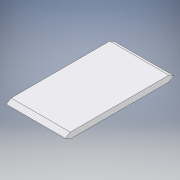
# Autodesk Inventor part: 雪弗板
Saved by Autodesk Inventor 2017 (Build 210142000, 142)
## iProperties
Part Number: 雪弗板
Material: 常规
Document SubType Name: Modeling
Designer: PANDA
Density: 1 g/cm^3
Appearance: 默认
Author: PANDA
Autodesk Inventor part; units mm, degrees
ref_plane "YZ Plane" through (0, 0, 0) normal (1, 0, 0) x (0, 1, 0)
ref_plane "XZ Plane" through (0, 0, 0) normal (0, 1, 0) x (-1, 0, 0)
ref_plane "XY Plane" through (0, 0, 0) normal (0, 0, 1) x (1, 0, 0)
sketch "草图1" plane through (0, 0, 0) normal (1, 0, 0) x (0, 1, 0)
  point P0 (0, 0)
sketch "草图6" plane through (0, 0, 0) normal (1, 0, 0) x (0, 1, 0)
  line L0 (275, 0) -> (250, 15)
  line L1 (250, 15) -> (-250, 15)
  line L2 (-250, 15) -> (-275, 0)
  line L3 (-275, 0) -> (-250, -15)
  line L4 (-250, -15) -> (250, -15)
  line L5 (250, -15) -> (275, 0)
  point P0 (0, 0)
  constraints: 12 end point, 3 parallel, 1 horizontal, 1 point on line
extrude "拉伸3" add sketch "草图6" along normal blind 300
